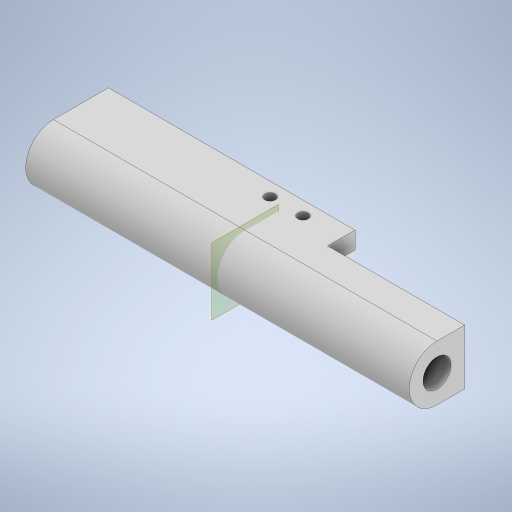
# Autodesk Inventor part: arm_connector
Saved by Autodesk Inventor 2024 (Build 280153000, 153)
## iProperties
Created: 2023-10-26
Part Number: arm_connector
Material: Generic
Document SubType Name: Modeling
Designer: dimademler
Density: 1 g/cm^3
Appearance: Default
Author: dimademler
Autodesk Inventor part; units mm, degrees
ref_plane "YZ Plane" through (0, 0, 0) normal (1, 0, 0) x (0, 1, 0)
ref_plane "XZ Plane" through (0, 0, 0) normal (0, 1, 0) x (-1, 0, 0)
ref_plane "XY Plane" through (0, 0, 0) normal (0, 0, 1) x (1, 0, 0)
sketch "Sketch1" plane through (0, 0, 0) normal (1, 0, 0) x (0, 1, 0)
  circle A0 centre (0, 0) radius 6.477
  circle A1 centre (0, 0) radius 12.827
  dimension "connector_inner_width" = 12.954
  dimension "connector_outerdiam" = 25.654
  constraints: 2 centre point, 2 coincident
  measures "connector_inner_width" diameter of A0
  measures "connector_outerdiam" diameter of A1
extrude "Extrusion1" add sketch "Sketch1" along normal blind 177.8
ref_plane "Work Plane1" through (88.9, 0, 0) normal (-1, 0, 0) x (0, 0, 1)
sketch "Sketch2" plane through (0, 0, 0) normal (-1, 0, 0) x (0, 0, 1)
  circle A0 centre (0, 0) radius 12.827 projected
  arc A1 (0, -12.827) -> (0, 12.827) centre (0, 0) ccw construction
  line L0 (-12.827, 0) -> (-12.827, 4.826)
  line L1 (-12.827, 4.826) -> (-25.527, 4.826)
  line L2 (-12.827, 4.826) -> (-12.827, 12.827) construction
  line L3 (-12.827, 0) -> (-12.827, -12.827)
  line L4 (-12.827, -12.827) -> (0, -12.827)
  line L5 (-12.827, 12.827) -> (0, 12.827)
  line L6 (-25.527, 4.826) -> (-25.527, 12.827)
  line L7 (-25.527, 12.827) -> (-12.827, 12.827)
  arc A2 (-12.827, 0) -> (0, -12.827) centre (0, 0) ccw
  arc A3 (0, 12.827) -> (-12.827, 0) centre (0, 0) ccw
  point P0 (-12.827, 0)
  point P1 (-12.827, 0)
  point P2 (0, -12.827)
  dimension "conector_tower_connection_thickness" = 4.826
  dimension "d5" = 12.7
  constraints: 16 end point, 6 point on circle, 5 tangent, 4 vertical, 3 centre point, 3 horizontal, 2 parallel, 1 coincident, 1 concentric
  measures "conector_tower_connection_thickness" distance of L0.start L0.end
  measures "d5" distance of L0.end L1.end
extrude "Extrusion2" add sketch "Sketch2" against normal blind 177.8 contours A0 L0 L1 L6 L7 L5 | L4 L3 A0
sketch "Sketch3" plane through (0, 4.826, -25.527) normal (0, -1, 0) x (1, 0, 0)
  line L0 (0, 12.7) -> (177.8, 12.7) projected
  line L1 (0, 0) -> (177.8, 0) projected
  line L2 (88.9, 0) -> (88.9, 12.7) construction
  line L3 (88.9, 0) -> (88.9, 12.7) construction
  line L4 (88.9, 6.35) -> (96.52, 6.35) construction
  circle A0 centre (96.52, 6.35) radius 2.413
  line L5 (88.9, 6.35) -> (81.28, 6.35) construction
  circle A1 centre (81.28, 6.35) radius 2.413
  point P0 (0, 25.527)
  dimension "d8" = 7.62
  dimension "d9" = 4.826
  constraints: 8 end point, 3 midpoint, 2 centre point, 2 coincident, 2 symmetric about line, 1 collinear, 1 horizontal, 1 other
  measures "d8" distance of L4.start L4.end
  measures "d9" diameter of A0
extrude "Extrusion3" cut sketch "Sketch3" against normal through all
sketch "Sketch4" plane through (0, -12.827, -12.827) normal (0, 0, -1) x (-1, 0, 0)
  line L0 (0, 0) -> (-177.8, 0) projected
  line L1 (0, 17.653) -> (-177.8, 17.653) projected
  line L2 (-88.9, 8.9535) -> (-38.1, 8.9535) construction
  line L3 (-177.8, 6.35) -> (-177.8, 19.304) projected
  line L4 (-177.8, 12.827) -> (0, 12.827) construction
  line L5 (-88.9, 12.827) -> (-139.7, 12.827)
  circle A0 centre (-139.7, 12.827) radius 2.413
  line L6 (-88.9, 0) -> (-88.9, 17.653) construction
  circle A1 centre (-38.1, 12.827) radius 2.413
  dimension "d14" = 50.8
  dimension "d15" = 4.826
  constraints: 8 end point, 4 midpoint, 2 centre point, 1 coincident, 1 horizontal, 1 point on line, 1 symmetric about line, 1 other
  measures "d14" distance of L5.start L5.end
  measures "d15" diameter of A0
extrude "Extrusion4" cut sketch "Sketch4" against normal blind 12.7
sketch "Sketch5" plane through (0, 4.826, -25.527) normal (0, -1, 0) x (1, 0, 0)
  line L0 (0, 12.7) -> (177.8, 12.7) projected
  line L1 (177.8, 12.7) -> (177.8, 0) projected
  line L2 (0, 0) -> (177.8, 0) projected
  circle A0 centre (96.52, 6.35) radius 2.413 projected
  line L3 (177.8, 0) -> (114.3, 0)
  line L4 (114.3, 0) -> (114.3, 12.7)
  line L5 (114.3, 12.7) -> (177.8, 12.7)
  point P0 (0, 25.527)
  dimension "d18" = 63.5
  constraints: 6 end point, 2 point on line, 1 collinear, 1 perpendicular
  measures "d18" distance of L1.end L3.end
extrude "Extrusion5" cut sketch "Sketch5" against normal blind 12.7 contours L0 L1 L2 L4
equation "\"d6\" = connector_width"
equation "\"connector_width\" = 177.8"
body "Solid1"
